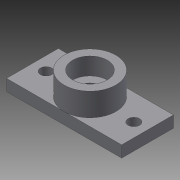
# Autodesk Inventor part: orczyk
Saved by Autodesk Inventor 2013 (Build 170138000, 138)
## iProperties
Created: 2014-04-23
Part Number: orczyk
Material: Generic
Document SubType Name: Modeling
Designer: Masta
Density: 1 g/cm^3
Author: Masta
Autodesk Inventor part; units mm, degrees
ref_plane "YZ Plane" through (0, 0, 0) normal (1, 0, 0) x (0, 1, 0)
ref_plane "XZ Plane" through (0, 0, 0) normal (0, 1, 0) x (-1, 0, 0)
ref_plane "XY Plane" through (0, 0, 0) normal (0, 0, 1) x (1, 0, 0)
sketch "Sketch1" plane through (0, 0, 0) normal (0, 0, 1) x (1, 0, 0)
  circle A0 centre (0, 0) radius 3
  circle A1 centre (0, 0) radius 4.5
  line L0 (0, 0) -> (7.62, 0) construction
  line L1 (0, 0) -> (-7.62, 0) construction
  line L2 (10, -4.5) -> (-10, -4.5)
  line L3 (-10, -4.5) -> (-10, 4.5)
  line L4 (-10, 4.5) -> (10, 4.5)
  line L5 (10, 4.5) -> (10, -4.5)
  line L6 (10, -4.5) -> (-10, 4.5) construction
  line L7 (-10, -4.5) -> (10, 4.5) construction
  circle A2 centre (0, 0) radius 1.5
  dimension "d0" = 6
  dimension "d1" = 9
  dimension "d2" = 7.62
  dimension "d3" = 7.62
  dimension "d4" = 20
  dimension "d5" = 9
  dimension "d8" = 3
  constraints: 16 end point, 5 coincident, 3 centre point, 3 equal length, 2 horizontal, 2 midpoint, 1 perpendicular
  measures "d0" diameter of A0
  measures "d1" diameter of A1
  measures "d2" distance of L0.start L0.end
  measures "d3" distance of L0.start L1.end
  measures "d4" distance of L3.end L4.end
  measures "d5" distance of L2.end L3.end
  measures "d8" diameter of A2
extrude "Extrusion1" add sketch "Sketch1" against normal blind 2 contours A1 | A1 L4 L5 L2 | A1 L2 L3 L4
extrude "Extrusion2" add sketch "Sketch1" along normal blind 1 contours A0 | A1
extrude "Extrusion3" add sketch "Sketch1" along normal blind 4 contours A1
hole "Hole1" at (-7.62, 0, 0) at (7.62, 0, 0) direction (0, 0, -1) diameter 2 end through all
body "Solid1"
